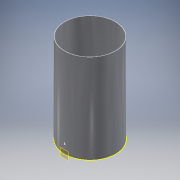
# Autodesk Inventor part: Water Jug
Saved by Autodesk Inventor 2018 (Build 220112000, 112)
## iProperties
Created: 2019-07-25
Part Number: Water Jug
Material: PC/ABS Plastic
Document SubType Name: Modeling
Designer: micha
Density: 0.357273 g/cm^3
Appearance: Smooth - White
Author: micha
Autodesk Inventor part; units mm, degrees
ref_plane "YZ Plane" through (0, 0, 0) normal (1, 0, 0) x (0, 1, 0)
ref_plane "XZ Plane" through (0, 0, 0) normal (0, 1, 0) x (-1, 0, 0)
ref_plane "XY Plane" through (0, 0, 0) normal (0, 0, 1) x (1, 0, 0)
sketch "Sketch1" plane through (0, 0, 0) normal (0, 1, 0) x (-1, 0, 0)
  circle A0 centre (0, 0) radius 73.025
  dimension "d0" = 146.05
  constraints: 1 centre point, 1 coincident
  measures "d0" diameter of A0
extrude "Extrusion1" add sketch "Sketch1" along normal blind 254
sketch "Sketch2" plane through (0, 254, 0) normal (0, 1, 0) x (1, 0, 0)
  circle A0 centre (0, 0) radius 73.025 projected
  circle A1 centre (0, 0) radius 71.4375
  dimension "d3" = 1.5875
  constraints: 1 centre point
  measures "d3" radial gap between concentric circles of A0 A1
extrude "Extrusion2" cut sketch "Sketch2" against normal blind 252.4125 contours A1
sketch "Sketch3" plane through (0, 0, 0) normal (0, -1, 0) x (1, 0, 0)
  circle A0 centre (0, 0) radius 73.025 projected
  point P0 (0, 73.025)
  constraints: 1 vertical alignment, 1 other
ref_plane "Work Plane1" through (0, 0, 73.025) normal (0, 0, 1) x (1, 0, 0)
sketch "Sketch4" plane through (0, 0, 73.025) normal (0, 0, 1) x (1, 0, 0)
  circle A0 centre (0, 25.4) radius 3.175
  point P0 (0, 0)
  dimension "d6" = 6.35
  dimension "d7" = 25.4
  constraints: 1 centre point
  measures "d6" diameter of A0
  measures "d7" distance of point (0, 0) A0.centre
extrude "Extrusion3" cut sketch "Sketch4" against normal blind 25.4
body "Solid1"
